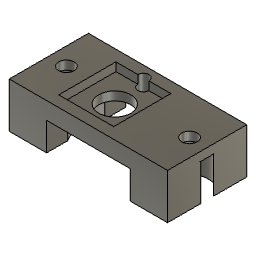
Encoder_block v4 (Autodesk Fusion 360 design; units mm, degrees)
Autodesk Fusion 360 part; units mm, degrees
sketch "Skizze1" plane through (0, 0, 0) normal (0, 0, 1) x (1, 0, 0)
  line L0 (18, -9) -> (-18, -9)
  line L1 (-18, -9) -> (-18, 9)
  line L2 (-18, 9) -> (18, 9)
  line L3 (18, 9) -> (18, -9)
  line L4 (18, -9) -> (-18, 9) construction
  line L5 (-18, -9) -> (18, 9) construction
  line L6 (-14, 14.295) -> (-14, -12) construction
  line L7 (14, 15.3346) -> (14, -11.7486) construction
  line L8 (-3, 14) -> (-3, -10) construction
  line L9 (-21.8783, 0) -> (29.3882, 0) construction
  circle A0 centre (-3, 0) radius 3.65
  circle A1 centre (-14, 0) radius 1.75
  circle A2 centre (14, 0) radius 1.75
  line L10 (-9.5, 9) -> (-9.5, -9)
  line L11 (9.5, 9) -> (9.5, -9)
  circle A3 centre (-3, 0) radius 7.75
  line L12 (3, -6.25) -> (-9, -6.25)
  line L13 (-9, -6.25) -> (-9, 6.25)
  line L14 (-9, 6.25) -> (3, 6.25)
  line L15 (3, 6.25) -> (3, -6.25)
  line L16 (3, -6.25) -> (-9, 6.25) construction
  line L17 (-9, -6.25) -> (3, 6.25) construction
  circle A4 centre (-14, 0) radius 4.25
  circle A5 centre (14, 0) radius 4.25
  point P0 (-6.65, 0)
  point P1 (-3, 0)
  dimension "d1" = 36
  dimension "d2" = 18
  dimension "d3" = 4
  dimension "d4" = 11
  dimension "d5" = 17
  dimension "d6" = 7.3
  dimension "d7" = 3.5
  dimension "d8" = 3.5
  dimension "d10" = 4.5
  dimension "d11" = 2.85
  dimension "d12" = 15.5
  dimension "d13" = 4.5
  dimension "d14" = 12
  dimension "d15" = 12.5
  dimension "d16" = 8.5
  dimension "d17" = 8.5
  constraint horizontal L0
  constraint perpendicular L0 L1
  constraint parallel L0 L2
  constraint parallel L1 L3
  constraint coincident L4 origin
  constraint coincident L5 origin
  constraint perpendicular L0 L6
  constraint perpendicular L0 L7
  constraint vertical L8
  constraint horizontal L9
  constraint coincident origin L9
  constraint coincident L9 P1
  constraint coincident L8 P1
  constraint coincident L9 A1.centre
  constraint coincident L6 A1.centre
  constraint coincident L9 A2.centre
  constraint coincident L7 A2.centre
  constraint coincident L2 L10.start
  constraint coincident L0 L10.end
  constraint perpendicular L0 L10
  constraint coincident L2 L11.start
  constraint coincident L0 L11.end
  constraint perpendicular L0 L11
  constraint coincident A0 P0
  constraint coincident L9 P0
  constraint concentric A0 A3
  constraint horizontal L12
  constraint perpendicular L12 L13
  constraint parallel L12 L14
  constraint parallel L13 L15
  constraint coincident L16 P1
  constraint coincident L17 P1
  constraint coincident P1 A0.centre
  constraint concentric A1 A4
  constraint concentric A2 A5
  measures "d1" distance of L1 L3
  measures "d2" distance of L0 L2
  measures "d3" distance of L1 L6
  measures "d4" distance of L6 L8
  measures "d5" distance of L7 L8
  measures "d6" diameter of A0
  measures "d7" diameter of A2
  measures "d8" diameter of A1
  measures "d10" distance of L7 L11
  measures "d11" distance of L10 P0
  measures "d12" diameter of A3
  measures "d13" distance of A1.centre L10
  measures "d14" distance of L13 L15
  measures "d15" distance of L12 L14
  measures "d16" diameter of A4
  measures "d17" diameter of A5
extrude "Extrusion1" add sketch "Skizze1" along normal blind 10.3 contours L0 L2 L3 L11 A5 | L0 L2 L10 L11 A3 L12 L13 L14 L15 | L3 A5 | L0 L1 L10 A3 A4 | L10 A3 A4 | L10 A3 L13 | L1 L2 L10 A3 A4 | L1 A3 A4 | A3 A4 | A3 L12 L13 L14 L15 | A3 L12 L13 | A3 L13 L14 | A3 L12 | A3 L14 | A3 L12 L15 | A3 L14 L15 | A3 L15 picked at (17.25, 0)
extrude "Extrusion2" cut sketch "Skizze1" along normal blind 8.3 contours L3 A5 | L1 A3 A4 | A3 A4 picked at (17.25, 0)
extrude "Extrusion3" cut sketch "Skizze1" along normal blind 6.4 contours L10 A3 A4 | L10 A3 L13 | A3 L12 L13 L14 L15 | A3 L12 | A3 L14 | A3 L15
extrude "Extrusion4" cut sketch "Skizze1" along normal blind 6.4 contours L0 L2 L10 L11 A3 L12 L13 L14 L15 | A3 L12 L13 | A3 L13 L14 | A3 L12 L15 | A3 L14 L15
sketch "Skizze2" plane through (0, 0, 10.3) normal (0, 0, 1) x (-1, 0, 0)
  circle A0 centre (-14, 0) radius 1.75
  circle A1 centre (14, 0) radius 1.75
  circle A2 centre (3, 0) radius 3.65
  line L0 (-18, -9) -> (18, -9)
  line L1 (18, -9) -> (18, 9)
  line L2 (18, 9) -> (-18, 9)
  line L3 (-18, 9) -> (-18, -9)
  line L4 (19.6534, 0) -> (-19.2741, 0) construction
  line L5 (3, -11.2204) -> (3, 11) construction
  line L6 (-3.25, 6.5) -> (9.25, 6.5)
  line L7 (9.25, 6.5) -> (9.25, -6.5)
  line L8 (9.25, -6.5) -> (-3.25, -6.5)
  line L9 (-3.25, -6.5) -> (-3.25, 6.5)
  line L10 (-3.25, 6.5) -> (9.25, -6.5) construction
  line L11 (9.25, 6.5) -> (-3.25, -6.5) construction
  circle A3 centre (3, -6.5) radius 1.25
  point P0 (3, 0)
  point P1 (3, 0)
  point P2 (3, -6.5)
  dimension "d26" = 13
  dimension "d27" = 12.5
  dimension "d30" = 2.5
  constraint perpendicular L3 L4
  constraint coincident L4 origin
  constraint perpendicular L2 L5
  constraint coincident L5 P1
  constraint horizontal L6
  constraint perpendicular L6 L7
  constraint parallel L6 L8
  constraint parallel L7 L9
  constraint coincident L10 P1
  constraint coincident L11 P1
  constraint coincident P1 P0
  constraint midpoint L8 P2
  constraint coincident P2 A3.centre
  measures "d26" distance of L6 L8
  measures "d27" distance of L7 L9
  measures "d30" diameter of A3
extrude "Extrusion5" cut sketch "Skizze2" against normal blind 1.92 contours L6 L7 L8 L9 A3 | L8 A3 picked at (3.3396, -6.2032)
extrude "Extrusion6" cut sketch "Skizze2" against normal blind 9 contours L8 A3 | L8 A3
